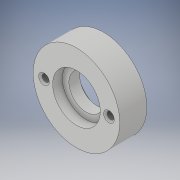
# Autodesk Inventor part: Корпус
Saved by Autodesk Inventor 2019.3 (Build 233278000, 278)
## iProperties
Created: 2020-04-02
Part Number: Корпус
Material: Типовые
Document SubType Name: Modeling
Designer: Admin
Density: 1 g/cm^3
Appearance: По умолчанию
Author: Admin
Autodesk Inventor part; units mm, degrees
ref_plane "YZ Plane" through (0, 0, 0) normal (1, 0, 0) x (0, 1, 0)
ref_plane "XZ Plane" through (0, 0, 0) normal (0, 1, 0) x (-1, 0, 0)
ref_plane "XY Plane" through (0, 0, 0) normal (0, 0, 1) x (1, 0, 0)
sketch "Эскиз1" plane through (0, 0, 0) normal (0, 0, 1) x (1, 0, 0)
  circle A0 centre (0, 0) radius 40
  dimension "d0" = 80
  constraints: 1 centre point, 1 coincident
  measures "d0" diameter of A0
extrude "Выдавливание1" add sketch "Эскиз1" along normal blind 25
sketch "Эскиз2" plane through (0, 0, 25) normal (0, 0, 1) x (1, 0, 0)
  point P0 (0, 0)
  point P1 (-30, 0)
  point P2 (30, 0)
  dimension "d3" = 30
  dimension "d4" = 60
  constraints: 2 horizontal alignment
  measures "d3" distance of point (0, 0) point (-30, 0)
  measures "d4" distance of point (30, 0) point (-30, 0)
hole "Отверстие1" at (-30, 0, 25) at (30, 0, 25) direction (0, 0, -1) diameter 6.647 depth 16.75 tip angle 120 thread size "M8x1.25" class "6H" standard "ANSI Metric M Profile"
chamfer "Фаска1" distance 1.6 angle 45 2 edges at (-30, 3.3235, 25) (30, 3.3235, 25)
sketch "Эскиз3" plane through (0, 0, 25) normal (0, 0, 1) x (1, 0, 0)
  circle A0 centre (0, 0) radius 22
  dimension "d15" = 44
  constraints: 1 centre point, 1 coincident
  measures "d15" diameter of A0
extrude "Выдавливание2" cut sketch "Эскиз3" against normal blind 9
sketch "Эскиз4" plane through (0, 0, 16) normal (0, 0, 1) x (1, 0, 0)
  circle A0 centre (0, 0) radius 16
  dimension "d18" = 32
  constraints: 1 centre point, 1 coincident
  measures "d18" diameter of A0
extrude "Выдавливание3" cut sketch "Эскиз4" against normal through all
sketch "Эскиз5" plane through (0, 0, 0) normal (0, 0, -1) x (-1, 0, 0)
  circle A0 centre (0, 0) radius 24
  dimension "d21" = 48
  constraints: 1 centre point, 1 coincident
  measures "d21" diameter of A0
extrude "Выдавливание4" cut sketch "Эскиз5" against normal blind 6
